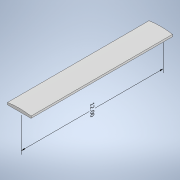
# Autodesk Inventor part: trussSupportForTube
Saved by Autodesk Inventor 2021.2 (Build 252289000, 289)
## iProperties
Created: 2021-02-11
Part Number: trussSupportForTube
Material: Generic
Document SubType Name: Modeling
Designer: robst
Density: 1 g/cm^3
Appearance: Default
Author: robst
Autodesk Inventor part; units mm, degrees
ref_plane "YZ Plane" through (0, 0, 0) normal (1, 0, 0) x (0, 1, 0)
ref_plane "XZ Plane" through (0, 0, 0) normal (0, 1, 0) x (-1, 0, 0)
ref_plane "XY Plane" through (0, 0, 0) normal (0, 0, 1) x (1, 0, 0)
sketch "Sketch1" plane through (0, 0, 0) normal (0, 0, 1) x (1, 0, 0)
  line L0 (0, 0) -> (25.4, 0)
  line L1 (0, 0) -> (-25.4, 0)
  arc A0 (25.4, 0) -> (-25.4, 0) centre (0, -156.7048) ccw
  line L2 (-25.4, 0) -> (-25.4, -4.3048)
  line L3 (-25.4, -4.3048) -> (25.4, -4.3048)
  line L4 (25.4, -4.3048) -> (25.4, 0)
  dimension "d0" = 25.4
  dimension "d1" = 25.4
  dimension "d2" = 158.75
  dimension "d3" = 6.35
  constraints: 10 end point, 2 horizontal, 2 perpendicular, 2 point on circle, 1 centre point, 1 vertical
  measures "d0" distance of L0.start L0.end
  measures "d1" distance of L0.start L1.end
  measures "d2" radius of A0
  measures "d3" distance edge to line of A0 L3
extrude "Extrusion1" add sketch "Sketch1" along normal mid plane 304.8
body "Solid1"
